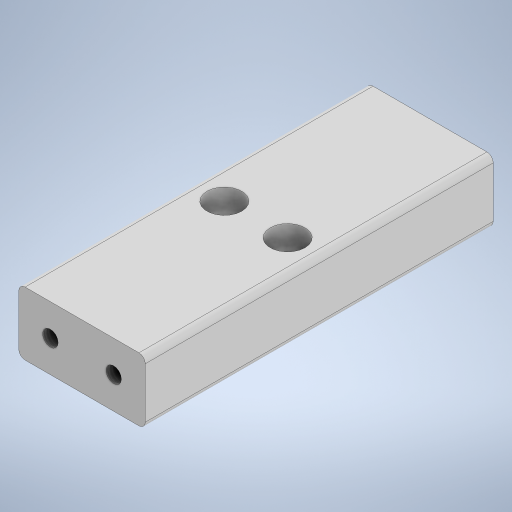
# Autodesk Inventor part: center_part
Saved by Autodesk Inventor 2024.3 (Build 283343010, 343A)
## iProperties
Created: 2025-07-19
Part Number: center_part
Material: 一般
Document SubType Name: Modeling
Designer: hikou
Density: 1 g/cm^3
Appearance: 既定
Author: hikou
Autodesk Inventor part; units mm, degrees
ref_plane "YZ Plane" through (0, 0, 0) normal (1, 0, 0) x (0, 1, 0)
ref_plane "XZ Plane" through (0, 0, 0) normal (0, 1, 0) x (-1, 0, 0)
ref_plane "XY Plane" through (0, 0, 0) normal (0, 0, 1) x (1, 0, 0)
sketch "スケッチ1" plane through (0, 0, 0) normal (0, 0, 1) x (1, 0, 0)
  line L0 (-10, 5) -> (10, 5)
  line L1 (10, 5) -> (10, -5)
  line L2 (10, -5) -> (-10, -5)
  line L3 (-10, -5) -> (-10, 5)
  line L4 (-10, 5) -> (10, -5) construction
  line L5 (10, 5) -> (-10, -5) construction
  point P0 (0, 0)
  dimension "d0" = 20
  dimension "d1" = 10
  constraints: 12 end point, 2 midpoint, 2 parallel, 1 horizontal, 1 perpendicular
  measures "d0" distance of L1.end L2.end
  measures "d1" distance of L0.end L1.end
extrude "押し出し1" add sketch "スケッチ1" along normal mid plane 55
sketch "スケッチ2" plane through (0, 0, 27.5) normal (0, 0, 1) x (1, 0, 0)
  line L0 (-10, -5) -> (10, -5) projected
  line L1 (-10, 5) -> (-10, -5) projected
  line L2 (10, -5) -> (10, 5) projected
  point P0 (0, 0)
  point P1 (-5, 0)
  point P2 (5, 0)
  dimension "d4" = 5
  dimension "d5" = 5
  dimension "d6" = 5
  dimension "d7" = 5
  measures "d4" distance from line of L0 point (-5, 0)
  measures "d5" distance from line of L1 point (-5, 0)
  measures "d6" distance from line of L0 point (5, 0)
  measures "d7" distance from line of L2 point (5, 0)
hole "穴1" at (-5, 0, 27.5) at (5, 0, 27.5) direction (0, 0, -1) diameter 2.459 depth 8.8 tip angle 118 thread size "M3x0.5" class "6H" standard "ISO Metric profile"
sketch "スケッチ3" plane through (0, 0, -27.5) normal (0, 0, -1) x (-1, 0, 0)
  line L0 (-10, -5) -> (10, -5) projected
  line L1 (10, -5) -> (10, 5) projected
  line L2 (10, 5) -> (-10, 5) projected
  line L3 (-10, 5) -> (-10, -5) projected
  circle A0 centre (-5, 0) radius 1.2295 projected
  circle A1 centre (5, 0) radius 1.2295 projected
  point P0 (0, 0)
  constraints: 2 coincident
hole "穴2" at (5, 0, -27.5) at (-5, 0, -27.5) direction (0, 0, 1) diameter 2.459 depth 8.8 tip angle 118 thread size "M3x0.5" class "6H" standard "ISO Metric profile"
sketch "スケッチ5" plane through (-10, 5, 27.5) normal (0, 1, 0) x (1, 0, 0)
  line L0 (20, 55) -> (20, 0) projected
  line L1 (0, 55) -> (20, 55) projected
  point P0 (10, 27.5)
  point P1 (15, 27.5)
  point P2 (5, 27.5)
  dimension "d22" = 5
  dimension "d23" = 10
  dimension "d24" = 27.5
  dimension "d25" = 27.5
  measures "d22" distance from line of L0 point (15, 27.5)
  measures "d23" distance of point (5, 27.5) point (15, 27.5)
  measures "d24" distance from line of L1 point (15, 27.5)
  measures "d25" distance from line of L1 point (5, 27.5)
hole "穴3" at (5, 5, 0) at (-5, 5, 0) direction (0, -1, 0) diameter 5.5 end through all
fillet "フィレット1" radius 1 4 edges at (-10, 5, 0) (10, 5, 0) (10, -5, 0) (-10, -5, 0)
equation "\"d5\" = d4"
equation "\"d6\" = d4"
equation "\"d7\" = d5"
equation "\"d25\" = d24"
